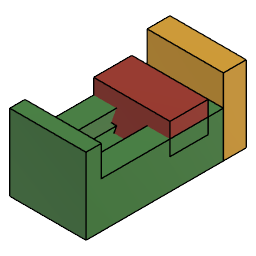
ex1 (Autodesk Fusion 360 design; units mm, degrees)
part number: 2026-03-30-18-39-52-591
part number: 2026-03-30-19-08-17-193
part number: 2026-03-30-19-08-24-188
part number: 2026-03-30-19-08-27-207
Autodesk Fusion 360 part; units mm, degrees
sketch "Sketch1" plane through (0, 0, 0) normal (0, 1, 0) x (1, 0, 0)
  line L0 (0, 0) -> (50, 0)
  line L1 (50, 0) -> (50, -50)
  line L2 (50, -50) -> (0, -50)
  line L3 (0, -50) -> (0, 0)
  line L4 (50, 0) -> (50, -30) construction
  line L5 (50, -30) -> (35, -30)
  line L6 (25, 0) -> (25, -15) construction
  line L7 (0, -30) -> (15, -30)
  line L8 (50, -15) -> (40, -15) construction
  line L9 (0, -15) -> (10, -15) construction
  line L10 (10, -15) -> (40, -15)
  line L11 (15, -30) -> (10, -15)
  line L12 (35, -30) -> (40, -15)
  line L13 (35, -30) -> (15, -30)
  dimension "d1" = 50
  dimension "d2" = 50
  dimension "d3" = 30
  dimension "d4" = 15
  dimension "d5" = 10
  dimension "d6" = 10
  dimension "d7" = 15
  dimension "d8" = 30
  dimension "d9" = 15.8114
  constraint horizontal L0
  constraint vertical L1
  constraint horizontal L2
  constraint vertical L3
  constraint coincident L0.start L3.end
  constraint perpendicular L0 L4
  constraint perpendicular L1 L5
  constraint midpoint L0 L6.start
  constraint perpendicular L0 L6
  constraint coincident L3 L7.start
  constraint perpendicular L3 L7
  constraint midpoint L4 L8.start
  constraint perpendicular L1 L8
  constraint coincident L3 L9.start
  constraint perpendicular L3 L9
  measures "d1" distance of L0.start L0.end
  measures "d2" distance of L0.start L2.end
  measures "d3" distance of L0.end L4.end
  measures "d4" distance of L7.start L7.end
  measures "d5" distance of L8.start L8.end
  measures "d6" distance of L9.start L9.end
  measures "d7" distance of L0 L9.end
  measures "d8" distance of L0 L7
  measures "d9" distance of L5.end L8.end
extrude "Extrude1" add sketch "Sketch1" along normal blind 10 contours L1 L2 L3 L5 L7 L13 | L10 L11 L12 L13 makes body 1
extrude "Extrude2" add sketch "Sketch1" along normal blind 90 contours L0 L1 L3 L5 L7 L10 L11 L12 bodies 1
extrude "Extrude3" add sketch "Sketch1" along normal blind 25 separate body contours L1 L2 L3 L5 L7 L13 | L10 L11 L12 L13 makes body 2
move_body "Move1" bodies 2 to x (1, 0, 0) y (0, 1, 0) z (0, 0, 1) at (-31.0805, 0, 27.7747)
extrude "Extrude4" add sketch "Sketch1" along normal blind 15 separate body contours L0 L1 L3 L5 L7 L10 L11 L12 | L1 L2 L3 L5 L7 L13 makes body 3
extrude "Extrude5" add sketch "Sketch1" along normal blind 25 contours L10 L11 L12 L13 bodies 3
move_body "Move2" bodies 2 to x (1, 0, 0) y (0, 1, 0) z (0, 0, 1) at (-6.8593, 0.6304, 19.3989)
move_body "Move3" bodies 3 to x (1, 0, 0) y (0, 1, 0) z (0, 0, 1) at (34.4399, -44.0515, 27.2123)
copy_body "Body->Comp1" bodies 1 removing the originals makes body 4 in component "Suport"
copy_body "Body->Comp2" bodies 2 removing the originals makes body 5 in component "Piesa sus"
copy_body "Body->Comp3" bodies 3 removing the originals makes body 6 in component "Piesa fata"
component "Suport" placed x (1, 0, 0) y (0, 1, 0) z (0, 0, 1) at (0, 0, 0)
component "Piesa sus" placed x (1, 0, 0) y (0, 1, 0) z (0, 0, 1) at (37.9397, 54.3696, -57.1736)
component "Piesa fata" placed x (-1, 0, 0) y (0, -1, 0) z (0, 0, 1) at (84.4399, 60.9485, -27.2123)
component "ex1" placed x (1, 0, 0) y (0, 1, 0) z (0, 0, 1) at (0, 0, 0) in component "Piesa fata"
named bodies: "Suport", "Piesa sus", "Piesa fata"
